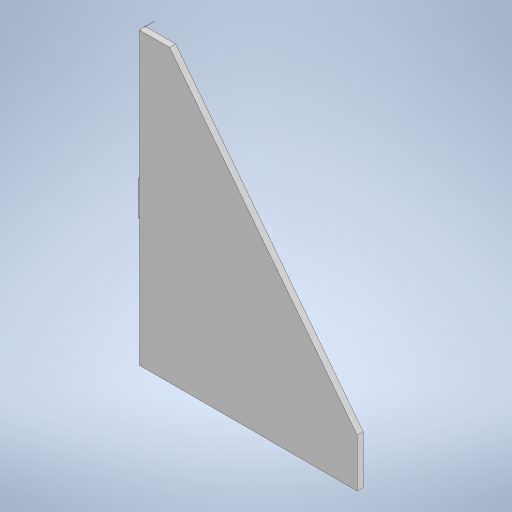
# Autodesk Inventor part: stock wall triangl
Saved by Autodesk Inventor 2023 (Build 270158000, 158)
## iProperties
Created: 2022-08-18
Part Number: stock wall triangl
Material: Generic
Document SubType Name: Modeling
Designer: rkant
Density: 1 g/cm^3
Appearance: Default
Author: rkant
Autodesk Inventor part; units mm, degrees
ref_plane "YZ Plane" through (0, 0, 0) normal (1, 0, 0) x (0, 1, 0)
ref_plane "XZ Plane" through (0, 0, 0) normal (0, 1, 0) x (-1, 0, 0)
ref_plane "XY Plane" through (0, 0, 0) normal (0, 0, 1) x (1, 0, 0)
sketch "Sketch1" plane through (0, 0, 0) normal (0, 0, 1) x (1, 0, 0)
  line L0 (457.2, -406.4) -> (457.2, -609.6)
  line L1 (457.2, -609.6) -> (-457.2, -609.6)
  line L2 (-457.2, -609.6) -> (-457.2, 609.6)
  line L3 (-457.2, 609.6) -> (-330.2, 609.6)
  line L4 (762.0015, 0.0045) -> (-761.9985, -0.0045) construction
  line L5 (457.2, -609.6) -> (-457.2, 609.6) construction
  line L6 (457.2, -406.4) -> (-330.2, 609.6)
  point P0 (0, 0)
  dimension "d0" = 681.5582
  dimension "d1" = 914.4
  dimension "d2" = 203.2
  dimension "d3" = 127
  dimension "d4" = 1219.2
  constraints: 14 end point, 2 parallel, 1 midpoint, 1 perpendicular, 1 point on line
  measures "d0" distance of L4.start L0.end
  measures "d1" distance of L1.end L0.end
  measures "d2" distance of L0.start L0.end
  measures "d3" distance of L3.end L2.end
  measures "d4" distance of L2.start L2.end
extrude "Extrusion1" add sketch "Sketch1" along normal blind 25.4
body "Solid1"
